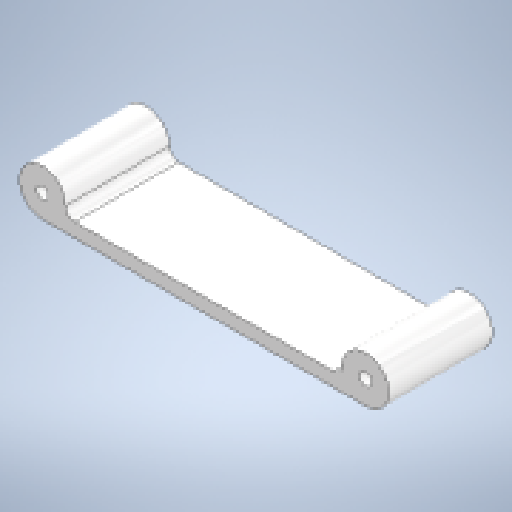
# Autodesk Inventor part: bad_huta
Saved by Autodesk Inventor 2025.1 (Build 291241000, 241)
## iProperties
Created: 2024-09-04
Part Number: bad_huta
Material: ABS プラスチック
Document SubType Name: Modeling
Designer: right
Density: 1.06 g/cm^3
Appearance: 滑らか - 黒
Mass: 6.34155 g
Surface Area: 49.7909 cm^2
Volume: 5.98259 cm^3
Author: right
Autodesk Inventor part; units mm, degrees
ref_plane "YZ Plane" through (0, 0, 0) normal (1, 0, 0) x (0, 1, 0)
ref_plane "XZ Plane" through (0, 0, 0) normal (0, 1, 0) x (-1, 0, 0)
ref_plane "XY Plane" through (0, 0, 0) normal (0, 0, 1) x (1, 0, 0)
sketch "スケッチ1" plane through (0, 0, 0) normal (0, 0, 1) x (1, 0, 0)
  circle A0 centre (-40, -15) radius 2 projected
  circle A1 centre (-40, -15) radius 1.3
  circle A2 centre (-40, -15) radius 4
  circle A3 centre (30, -15) radius 2 projected
  circle A4 centre (30, -15) radius 1.3
  circle A5 centre (30, -15) radius 4
  line L0 (-36.5359, -17) -> (26.5359, -17)
  line L1 (33, -12.0514) -> (33, -20) projected
  line L2 (-43, 18) -> (33, 18) projected
  line L3 (-43, -20) -> (-43, 18) projected
  line L4 (-43, -20) -> (33, -20) projected
  circle A6 centre (30, -15) radius 2 projected
  circle A7 centre (-40, -15) radius 2 projected
  circle A8 centre (48, 10) radius 1.3 projected
  line L5 (49.2255, 7.2617) -> (41.3517, 3.7378) projected
  arc A9 (49.2255, 7.2617) -> (49.2255, 12.7383) centre (48, 10) ccw projected
  line L6 (33, 20) -> (49.2255, 12.7383) projected
  line L7 (33, 18) -> (33, 20) projected
  line L8 (12.9502, 12.2111) -> (-6.1056, 2.6833) projected
  arc A10 (-7.8944, 2.6833) -> (-6.1056, 2.6833) centre (-7, 4.4721) ccw projected
  line L9 (-7.8944, 2.6833) -> (-26.9502, 12.2111) projected
  arc A11 (-26.0557, 16) -> (-26.9502, 12.2111) centre (-26.0557, 14) ccw projected
  line L10 (-26.0557, 16) -> (12.0557, 16) projected
  arc A12 (12.9502, 12.2111) -> (12.0557, 16) centre (12.0557, 14) ccw projected
  line L11 (-30.9502, -14.2111) -> (-7.8944, -2.6833) projected
  arc A13 (-6.1056, -2.6833) -> (-7.8944, -2.6833) centre (-7, -4.4721) ccw projected
  line L12 (-6.1056, -2.6833) -> (16.9502, -14.2111) projected
  arc A14 (16.0557, -18) -> (16.9502, -14.2111) centre (16.0557, -16) ccw projected
  line L13 (16.0557, -18) -> (-30.0557, -18) projected
  arc A15 (-30.9502, -14.2111) -> (-30.0557, -18) centre (-30.0557, -16) ccw projected
  arc A16 (-15.0498, -1.7889) -> (-15.0498, 1.7889) centre (-15.9443, 0) ccw projected
  line L14 (-15.0498, -1.7889) -> (-36.5067, -12.5173) projected
  arc A17 (-38.4407, -12.4371) -> (-36.5067, -12.5173) centre (-37.4012, -10.7285) ccw projected
  arc A18 (-38.4407, -12.4371) -> (-39.4, -12.0606) centre (-40, -15) ccw projected
  arc A19 (-41, -10.101) -> (-39.4, -12.0606) centre (-39, -10.101) ccw projected
  line L15 (-41, -10.101) -> (-41, 11.5279) projected
  arc A20 (-38.1056, 13.3167) -> (-41, 11.5279) centre (-39, 11.5279) ccw projected
  line L16 (-38.1056, 13.3167) -> (-15.0498, 1.7889) projected
  line L17 (1.0498, 1.7889) -> (28.1056, 15.3167) projected
  arc A21 (31, 13.5279) -> (28.1056, 15.3167) centre (29, 13.5279) ccw projected
  line L18 (31, 13.5279) -> (31, -10.101) projected
  arc A22 (29.4, -12.0606) -> (31, -10.101) centre (29, -10.101) ccw projected
  arc A23 (29.4, -12.0606) -> (27.5909, -13.2122) centre (30, -15) ccw projected
  arc A24 (25.0904, -13.8091) -> (27.5909, -13.2122) centre (25.9849, -12.0203) ccw projected
  line L19 (25.0904, -13.8091) -> (1.0498, -1.7889) projected
  arc A25 (1.0498, 1.7889) -> (1.0498, -1.7889) centre (1.9443, 0) ccw projected
  arc A26 (45.0001, 10.0279) -> (45.0001, 9.9721) centre (48, 10) ccw projected
  arc A27 (43.8172, 8.128) -> (45.0001, 9.9721) centre (43.0002, 9.9535) ccw projected
  line L20 (43.8172, 8.128) -> (38.817, 5.8902) projected
  arc A28 (36, 7.7157) -> (38.817, 5.8902) centre (38, 7.7157) ccw projected
  line L21 (36, 7.7157) -> (36, 12.2843) projected
  arc A29 (38.817, 14.1098) -> (36, 12.2843) centre (38, 12.2843) ccw projected
  line L22 (38.817, 14.1098) -> (43.8172, 11.872) projected
  arc A30 (45.0001, 10.0279) -> (43.8172, 11.872) centre (43.0002, 10.0465) ccw projected
  spline S0 degree 3 poles (41.3517, 3.7378) (39.988, 3.1275) (38.7646, 2.2569) (36.3724, -0.2353) (35.577, -1.7516) (34.5201, -4.2662) (34.1294, -5.7212) (33.5024, -8.8036) (33.2459, -10.4611) (33.0027, -12.0338) (33.0014, -12.0426) (33, -12.0514) knots 0 0 0 0 0.448208 0.448208 1.03384 1.03384 1.722667 1.722667 2.343954 2.343954 2.347451 2.347451 2.347451 2.347451 projected
  point P0 (0, 0)
  point P1 (-40, -20)
  point P2 (30, -20)
  point P3 (33, -17.6458)
  point P4 (-43, -17.6458)
  point P5 (-43, -12.3542)
  point P6 (33, -12.3542)
  dimension "d1" = 8
  dimension "d3" = 8
  dimension "d0" = 2.6
  dimension "d2" = 2.6
  dimension "d4" = 3
  constraints: 4 coincident, 2 centre point, 2 end point, 1 horizontal, 6 other
  measures "d0" diameter of A1
  measures "d2" diameter of A4
  measures "d4" distance between parallel lines of L0 L4
ref_plane "作業平面1" through (-35, -20, 20) normal (0, 0, -1) x (0, 1, 0)
ref_plane "作業平面2" through (-35, -20, 24.5) normal (0, 0, -1) x (0, 1, 0)
ref_plane "作業平面3" through (-49.856, -31.0995, 22.5) normal (0, 0, -1) x (0, 1, 0)
extrude "押し出し1" add sketch "スケッチ1" along normal up to surface (22.5 mm away) contours A0 | A2 L3 A19 A18 A17 | L0 A15 L13 A14 A5 L1 L4 L3 A2 | A2 L3 | L0 A14 L13 A15 | A17 A18 A19 A2 | A5 A24 A23 A22 L1 | L1 A5 | A5 A22 A23 A24 | A3
fillet "フィレット1" radius 2 2 edges at (-36.5359, -17, 11.25) (26.5359, -17, 11.25)
sketch "スケッチ2" plane through (-40, -20, 0) normal (0, -1, 0) x (1, 0, 0)
  line L0 (-3, 22.5) -> (73, 22.5) projected
  line L1 (-3, 0) -> (73, 0) projected
  line L2 (68, 20.5) -> (2, 20.5)
  line L3 (2, 20.5) -> (2, 2)
  line L4 (2, 2) -> (68, 2)
  line L5 (68, 2) -> (68, 20.5)
  line L6 (0, 22.5) -> (70, 0) construction
  line L7 (35, 22.5) -> (35, 0) construction
  line L8 (0, 21.4496) -> (66.7321, 0)
  line L9 (0.612, 23.3537) -> (67.3441, 1.9041)
  line L10 (70, 21.4496) -> (3.2679, 0)
  line L11 (69.388, 23.3537) -> (2.6559, 1.9041)
  line L12 (-3, 0) -> (-3, 22.5) projected
  line L13 (73, 0) -> (73, 22.5) projected
  point P0 (40, 0)
  point P1 (67.0457, 20.5)
  point P2 (38.2679, 11.25)
  point P3 (67.0457, 2)
  point P4 (35, 10.1996)
  point P5 (9.4901, 2)
  point P6 (60.5099, 2)
  point P7 (35, 12.3004)
  point P8 (60.5099, 20.5)
  point P9 (9.4901, 20.5)
  point P10 (2.9543, 2)
  point P11 (31.7321, 11.25)
  point P12 (2.9543, 20.5)
  dimension "d8" = 2
  dimension "d9" = 1
  constraints: 20 end point, 6 symmetric about line, 2 midpoint, 1 parallel, 1 point on line
  measures "d8" distance between parallel lines of L0 L2
  measures "d9" distance between parallel lines of L8 L6
extrude "押し出し2" cut sketch "スケッチ2" against normal blind 1 contours L2 L11 L9 | L8 L11 L4 L3 L2 | L10 L8 L4 | L2 L5 L4 L9 L10
fillet "フィレット2" radius 2 16 edges at (-38, -19.5, 20.5) (-37.0457, -19.5, 20.5) (-30.5099, -19.5, 20.5) (-5, -19.5, 12.3004) (-8.2679, -19.5, 11.25) (-5, -19.5, 10.1996) (-1.7321, -19.5, 11.25) (20.5099, -19.5, 20.5) (28, -19.5, 20.5) (27.0457, -19.5, 20.5) (28, -19.5, 2) (27.0457, -19.5, 2) (20.5099, -19.5, 2) (-30.5099, -19.5, 2) (-38, -19.5, 2) (-37.0457, -19.5, 2)
fillet "フィレット3" radius 2 24 edges at (-37.1785, -19, 19.6799) (-24.7904, -19, 16.5608) (-12.8036, -19, 11.25) (-24.7904, -19, 5.9392) (-37.1785, -19, 2.8201) (-38, -19, 11.25) (9.7278, -19, 18.8097) (1.988, -19, 14.5465) (-5, -19, 12.4012) (-11.988, -19, 14.5465) (-19.7278, -19, 18.8097) (-5, -19, 20.5) (9.7278, -19, 3.6903) (-5, -19, 2) (-19.7278, -19, 3.6903) (-11.988, -19, 7.9535) (-5, -19, 10.0988) (1.988, -19, 7.9535) (27.1785, -19, 19.6799) (28, -19, 11.25) (27.1785, -19, 2.8201) (14.7904, -19, 5.9392) (2.8036, -19, 11.25) (14.7904, -19, 16.5608)
fillet "フィレット4" radius 2 4 edges at (-43, -20, 11.25) (-43, -17.6458, 11.25) (33, -20, 11.25) (33, -17.6458, 11.25)
equation "\"d3\" = d1"
